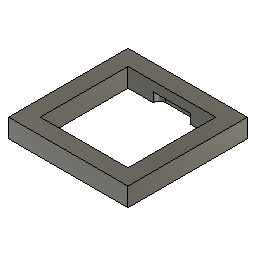
1U v2 (Autodesk Fusion 360 design; units mm, degrees)
Autodesk Fusion 360 part; units mm, degrees
sketch "スケッチ1" plane through (0, 0, 0) normal (0, 0, 1) x (1, 0, 0)
  line L0 (7, -7) -> (-7, -7)
  line L1 (-7, -7) -> (-7, 7)
  line L2 (-7, 7) -> (7, 7)
  line L3 (7, 7) -> (7, -7)
  line L4 (9.525, -9.525) -> (-9.525, -9.525)
  line L5 (-9.525, -9.525) -> (-9.525, 9.525)
  line L6 (-9.525, 9.525) -> (9.525, 9.525)
  line L7 (9.525, 9.525) -> (9.525, -9.525)
  line L8 (3, 7) -> (3, 7)
  line L9 (-3, 7) -> (-3, 7)
  line L10 (-2, 8) -> (2, 8)
  line L11 (3, -7) -> (3, -7)
  line L12 (2, -8) -> (-2, -8)
  line L13 (-3, -7) -> (-3, -7)
  arc A0 (2, -8) -> (3, -7) centre (2, -7) ccw
  arc A1 (-3, -7) -> (-2, -8) centre (-2, -7) ccw
  arc A2 (3, 7) -> (2, 8) centre (2, 7) ccw
  arc A3 (-2, 8) -> (-3, 7) centre (-2, 7) ccw
  dimension "d8" = 1
  constraint horizontal L0
  constraint perpendicular L0 L1
  constraint parallel L0 L2
  constraint parallel L1 L3
  constraint horizontal L4
  constraint perpendicular L4 L5
  constraint parallel L4 L6
  constraint parallel L5 L7
  constraint coincident L2 L8.start
  constraint coincident L2 L9.start
  constraint coincident L0 L11.start
  constraint coincident L0 L13.start
  constraint tangent L12 A0
  constraint tangent L12 A1
  constraint equal A0 A1
  constraint tangent L10 A2
  constraint equal A0 A2
  constraint tangent L10 A3
  constraint equal A0 A3
  measures "d8" radius of A0
extrude "押し出し1" add sketch "スケッチ1" along normal blind 3
extrude "押し出し2" add sketch "スケッチ1" along normal blind 1.5 from surface at 1.5 contours L0 L12 A0 A1 | L2 L10 A2 A3
